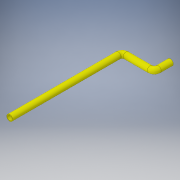
# Autodesk Inventor part: ABS Arm
Saved by Autodesk Inventor 2016 (Build 200138000, 138)
## iProperties
Created: 2015-07-12
Part Number: ABS Arm
Material: ABS Plastic
Document SubType Name: Modeling
Designer: steele
Density: 1.06 g/cm^3
Appearance: Smooth - Yellow
Author: steele
Autodesk Inventor part; units mm, degrees
ref_plane "YZ Plane" through (0, 0, 0) normal (1, 0, 0) x (0, 1, 0)
ref_plane "XZ Plane" through (0, 0, 0) normal (0, 1, 0) x (-1, 0, 0)
ref_plane "XY Plane" through (0, 0, 0) normal (0, 0, 1) x (1, 0, 0)
sketch "Sketch1" plane through (0, 0, 0) normal (0, 1, 0) x (-1, 0, 0)
  line L0 (0, 0) -> (0, 38.1)
  line L1 (12.7, 50.8) -> (88.9, 50.8)
  line L2 (101.6, 63.5) -> (101.6, 406.4)
  arc A0 (88.9, 50.8) -> (101.6, 63.5) centre (88.9, 63.5) ccw
  arc A1 (12.7, 50.8) -> (0, 38.1) centre (12.7, 38.1) ccw
  point P0 (0, 50.8)
  point P1 (101.6, 50.8)
  dimension "short" = 50.8
  dimension "right" = 101.6
  dimension "long" = 355.6
  dimension "turn_radisu" = 12.7
  dimension "d10" = 12.7
  constraints: 6 end point, 4 point on circle, 4 point on line, 4 tangent, 2 centre point, 2 perpendicular, 1 vertical
  measures "short" distance of L0.start point (0, 50.8)
  measures "right" distance of point (0, 50.8) point (101.6, 50.8)
  measures "long" distance of point (101.6, 50.8) L2.end
  measures "turn_radisu" radius of A0
  measures "d10" radius of A1
sketch "Sketch2" plane through (0, 0, 0) normal (0, 0, 1) x (1, 0, 0)
  circle A0 centre (0, 0) radius 9.525
  circle A1 centre (0, 0) radius 7.62
  dimension "outside_diamter" = 19.05
  dimension "inside_diameter" = 15.24
  constraints: 2 centre point, 2 coincident
  measures "outside_diamter" diameter of A0
  measures "inside_diameter" diameter of A1
sweep "Sweep2" add profiles "Sketch2" path "Sketch1" path curves L0 A1 L1 A0 L2
body "Solid2"
